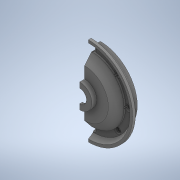
# Autodesk Inventor part: rotor-back-lid
Saved by Autodesk Inventor 2022 (Build 260153000, 153)
## iProperties
Created: 2025-01-14
Part Number: rotor-back-lid
Material: Generic
Document SubType Name: Modeling
Designer: Kostic
Density: 1 g/cm^3
Appearance: Default
Author: Kostic
Autodesk Inventor part; units mm, degrees
ref_plane "YZ Plane" through (0, 0, 0) normal (1, 0, 0) x (0, 1, 0)
ref_plane "XZ Plane" through (0, 0, 0) normal (0, 1, 0) x (-1, 0, 0)
ref_plane "XY Plane" through (0, 0, 0) normal (0, 0, 1) x (1, 0, 0)
sketch "Sketch1" plane through (0, 0, 0) normal (0, 0, 1) x (1, 0, 0)
  circle A0 centre (0, 0) radius 82
  dimension "d0" = 164
  constraints: 1 centre point, 1 coincident
  measures "d0" diameter of A0
extrude "Extrusion1" add sketch "Sketch1" along normal blind 38
sketch "Sketch2" plane through (0, 0, 38) normal (0, 0, 1) x (1, 0, 0)
  circle A0 centre (0, 0) radius 22.5
  circle A1 centre (0, 0) radius 82 projected
  dimension "d3" = 45
  constraints: 1 centre point, 1 coincident
  measures "d3" diameter of A0
extrude "Extrusion2" cut sketch "Sketch2" against normal blind 9
sketch "Sketch3" plane through (0, 0, 29) normal (0, 0, 1) x (1, 0, 0)
  circle A0 centre (0, 0) radius 82 projected
  circle A1 centre (0, 0) radius 60
  circle A2 centre (0, 0) radius 22.5 projected
  circle A3 centre (0, 0) radius 71
  dimension "d6" = 120
  dimension "d9" = 142
  constraints: 2 centre point, 2 coincident
  measures "d6" diameter of A1
  measures "d9" diameter of A3
extrude "Extrusion3" cut sketch "Sketch3" against normal blind 16 contours A3
move faces "Move1" translate (0, 0, -7) faces at (-38.9832, -67.6974, 29)
chamfer "Chamfer1" distance 6 distance2 9 1 edges at (-71, 0, 22) measured on face at (-38.9832, 67.6974, 22)
chamfer "Chamfer2" distance 16 distance2 13 1 edges at (-60, 0, 29) measured on face at (-44.5807, -15.7933, 29)
sketch "Sketch4" plane through (0, 0, 0) normal (0, 0, -1) x (-1, 0, 0)
  circle A0 centre (0, 0) radius 75
  circle A1 centre (0, 0) radius 82 projected
  dimension "d19" = 150
  constraints: 1 centre point, 1 coincident
  measures "d19" diameter of A0
extrude "Extrusion4" cut sketch "Sketch4" against normal blind 17
sketch "Sketch5" plane through (0, 0, 0) normal (0, 0, -1) x (-1, 0, 0)
  circle A0 centre (0, 0) radius 75 projected
  circle A1 centre (0, 0) radius 68.5
  dimension "d22" = 137
  constraints: 1 centre point, 1 coincident
  measures "d22" diameter of A1
extrude "Extrusion5" cut sketch "Sketch5" against normal blind 9
fillet "Fillet1" radius 4 2 edges at (75, 0, 9) (75, 0, 17)
fillet "Fillet2" radius 2 1 edges at (68.5, 0, 9)
sketch "Sketch6" plane through (0, 0, 0) normal (0, 0, -1) x (-1, 0, 0)
  circle A0 centre (0, 0) radius 68.5 projected
  circle A1 centre (0, 0) radius 58.7
  dimension "d30" = 117.4
  constraints: 1 centre point, 1 coincident
  measures "d30" diameter of A1
extrude "Extrusion6" cut sketch "Sketch6" against normal blind 15 contours A1
sketch "Sketch7" plane through (0, 0, 15) normal (0, 0, -1) x (-1, 0, 0)
  circle A0 centre (0, 0) radius 44
  dimension "d33" = 88
  constraints: 1 centre point, 1 coincident
  measures "d33" diameter of A0
extrude "Extrusion7" cut sketch "Sketch7" against normal blind 11
chamfer "Chamfer4" distance 13 distance2 11 1 edges at (44, 0, 15) measured on face at (-53.4856, -3.4938, 15)
sketch "Sketch8" plane through (0, 0, 26) normal (0, 0, -1) x (-1, 0, 0)
  circle A0 centre (0, 0) radius 21.5
  dimension "d39" = 43
  constraints: 1 centre point, 1 coincident
  measures "d39" diameter of A0
extrude "Extrusion8" add sketch "Sketch8" along normal blind 3
sketch "Sketch9" plane through (0, 0, 23) normal (0, 0, -1) x (-1, 0, 0)
  circle A0 centre (0, 0) radius 17.5
  dimension "d42" = 35
  constraints: 1 centre point, 1 coincident
  measures "d42" diameter of A0
extrude "Extrusion9" cut sketch "Sketch9" against normal blind 10
sketch "Sketch10" plane through (0, 0, 33) normal (0, 0, -1) x (-1, 0, 0)
  circle A0 centre (0, 0) radius 14
  dimension "d45" = 28
  constraints: 1 centre point, 1 coincident
  measures "d45" diameter of A0
extrude "Extrusion10" cut sketch "Sketch10" against normal blind 0.5
sketch "Sketch11" plane through (0, 0, 33.5) normal (0, 0, -1) x (-1, 0, 0)
  circle A0 centre (0, 0) radius 12.5
  dimension "d48" = 25
  constraints: 1 centre point, 1 coincident
  measures "d48" diameter of A0
extrude "Extrusion11" cut sketch "Sketch11" against normal blind 11
sketch "Sketch12" plane through (0, 0, 29) normal (0, 0, 1) x (1, 0, 0)
  circle A0 centre (0, 0) radius 12.5 projected
  line L0 (0, 0) -> (64, 0)
  dimension "d51" = 64
  constraints: 2 end point, 1 horizontal
  measures "d51" distance of L0.start L0.end
hole "Hole1" at (64, 0, 29) direction (0, 0, -1) diameter 4.2 end through all counterbore diameter 8.6 counterbore depth 20
fillet "Fillet3" radius 2 4 edges at (67.5397, 2.4414, 13) (61.5586, -3.5397, 13) (59.9805, 1.5277, 14.5) (59.9805, -1.5277, 14.5)
pattern_circular "Circular Pattern1" count 8 over 360 about axis through (0, 0, 29) along (0, 0, -1) of "Hole1", "Fillet3"
body "Solid1"
